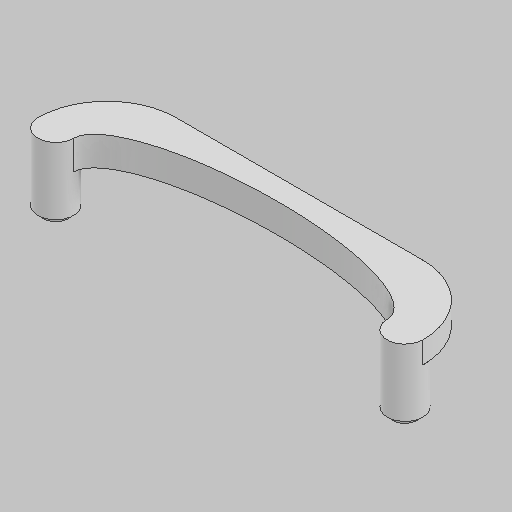
# Autodesk Inventor part: bumper
Saved by Autodesk Inventor 2026 (Build 300175000, 175)
## iProperties
Created: 2026-07-11
Part Number: bumper
Material: Generic
Document SubType Name: Modeling
Designer: admin
Density: 1 g/cm^3
Appearance: Default
Author: admin
Autodesk Inventor part; units mm, degrees
ref_plane "YZ Plane" through (0, 0, 0) normal (1, 0, 0) x (0, 1, 0)
ref_plane "XZ Plane" through (0, 0, 0) normal (0, 1, 0) x (-1, 0, 0)
ref_plane "XY Plane" through (0, 0, 0) normal (0, 0, 1) x (1, 0, 0)
sketch "Эскиз1" plane through (0, 0, 0) normal (0, 1, 0) x (-1, 0, 0)
  line L0 (0, -1.5) -> (0, 1.5)
  circle A0 centre (24, 8) radius 2.45
  ellipse E0 centre (0, 8) end of major axis (21.55, 8) minor radius 6.5
  line L1 (0, -1.5) -> (16.95, -1.5)
  arc A1 (16.95, -1.5) -> (26.45, 8) centre (16.95, 8) ccw
  point P0 (0, 0)
  point P1 (0, 0)
  point P2 (21.55, 8)
  dimension "d0" = 4.9
  dimension "d1" = 48
  dimension "d2" = 8
  dimension "d3" = 3
  constraints: 4 end point, 2 horizontal alignment, 2 point on circle, 1 centre point, 1 coincident, 1 horizontal, 1 midpoint, 1 tangent, 1 vertical, 1 vertical alignment, 7 other
  measures "d1" diameter of point (24, 8) L0
  measures "d2" vertical distance of point (24, 8) point (0, 0)
  measures "d3" distance of L0.start L0.end
extrude "Выдавливание1" add sketch "Эскиз1" along normal blind 4 contours L0 E0 A0 A1 L1 | A0
extrude "Выдавливание2" add sketch "Эскиз1" against normal blind 6 contours A0
mirror "Зеркальное отражение1" about plane through (0, 0, 1.5) normal (1, 0, 0)
chamfer "Фаска1" distance 1 angle 45 3 edges at (0, 0, -1.5) (23.6675, 0, 1.2825) (-23.6675, 0, 1.2825)
chamfer "Фаска2" distance 0.8 angle 45 2 edges at (-21.55, -6, 8) (21.55, -6, 8)
